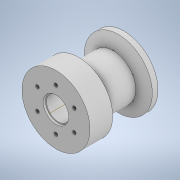
# Autodesk Inventor part: pulleyForRoundAdapter
Saved by Autodesk Inventor 2020.2 (Build 242310000, 310)
## iProperties
Created: 2020-02-15
Part Number: pulleyForRoundAdapter
Material: Generic
Document SubType Name: Modeling
Designer: robst
Density: 1 g/cm^3
Appearance: Default
Author: robst
Autodesk Inventor part; units mm, degrees
ref_plane "YZ Plane" through (0, 0, 0) normal (1, 0, 0) x (0, 1, 0)
ref_plane "XZ Plane" through (0, 0, 0) normal (0, 1, 0) x (-1, 0, 0)
ref_plane "XY Plane" through (0, 0, 0) normal (0, 0, 1) x (1, 0, 0)
sketch "Sketch1" plane through (0, 0, 0) normal (0, 0, 1) x (1, 0, 0)
  circle A0 centre (0, 0) radius 25.4
  dimension "d0" = 50.8
  constraints: 2 coincident, 1 centre point
  measures "d0" diameter of A0
extrude "Extrusion1" add sketch "Sketch1" along normal mid plane 76.2
sketch "Sketch3" plane through (0, 0, 0) normal (1, 0, 0) x (0, 1, 0)
  line L0 (25.4, 38.1) -> (-25.4, 38.1) projected
  line L1 (25.4, 38.1) -> (38.1, 38.1)
  line L2 (25.4, -38.1) -> (25.4, 38.1) projected
  line L3 (0, -53.34) -> (0, 53.34) projected
  line L4 (38.1, 38.1) -> (38.1, 12.7)
  line L5 (38.1, 12.7) -> (24.2886, 6.2597)
  line L6 (24.2886, 6.2597) -> (25.4, 6.7779)
  line L7 (25.4, -38.1) -> (25.4, 38.1) projected
  point P0 (0, 0)
  point P1 (25.4, 19.4779)
  point P2 (25.4, 6.7779)
  point P3 (25.4, 6.7779)
  dimension "d9" = 12.7
  dimension "d12" = 25.4
  dimension "d13" = 115
  constraints: 8 end point, 2 point on line, 1 collinear, 1 horizontal, 1 vertical
  measures "d9" distance of L0.start L1.end
  measures "d12" distance of L1.end L4.end
  measures "d13" angle of L4 L5
revolve "Revolution1" add sketch "Sketch3" angle 360 about axis through (0, 0, -10) along (0, 0, 1)
sketch "Sketch4" plane through (0, 0, 0) normal (1, 0, 0) x (0, 1, 0)
  line L0 (25.4, -38.1) -> (25.4, 6.7779) projected
  line L1 (-25.4, -38.1) -> (25.4, -38.1) projected
  line L2 (25.4, -38.1) -> (38.1, -38.1)
  line L3 (38.1, -38.1) -> (38.1, -31.75)
  line L4 (38.1, -31.75) -> (24.8707, -25.5811)
  line L5 (0, -46.9275) -> (0, 14.8652) projected
  line L6 (24.8707, -25.5811) -> (25.4, -25.8279)
  line L7 (25.4, -38.1) -> (25.4, 6.7779) projected
  point P0 (0, 0)
  dimension "d14" = 12.7
  dimension "d15" = 6.35
  dimension "d16" = 115
  constraints: 8 end point, 1 collinear, 1 horizontal, 1 perpendicular, 1 point on line
  measures "d14" distance of L0.start L2.end
  measures "d15" distance of L2.end L3.end
  measures "d16" angle of L4 L3
revolve "Revolution2" add sketch "Sketch4" angle 360 about axis through (0, 0, -10) along (0, 0, 1)
sketch "Sketch5" plane through (0, 0, 38.1) normal (0, 0, 1) x (1, 0, 0)
  circle A0 centre (0, 0) radius 13.0969
  dimension "d18" = 26.1938
  constraints: 1 centre point, 1 coincident
  measures "d18" diameter of A0
extrude "Extrusion4" cut sketch "Sketch5" against normal blind 25.4
sketch "Sketch6" plane through (0, 0, 38.1) normal (0, 0, 1) x (1, 0, 0)
  circle A0 centre (0, 0) radius 14.2875
  dimension "d21" = 28.575
  constraints: 1 centre point, 1 coincident
  measures "d21" diameter of A0
extrude "Extrusion5" cut sketch "Sketch6" against normal blind 2.54
mirror "Mirror2" about plane through (0, 0, 0) normal (0, 0, 1) of "Extrusion5", "Extrusion4"
sketch "Sketch8" plane through (0, 0, 38.1) normal (0, 0, 1) x (1, 0, 0)
  point P0 (0, 0)
  point P1 (0, 23.8125)
  point P2 (-20.6222, 11.9063)
  point P3 (0, 0)
  point P4 (-20.6222, -11.9062)
  point P5 (0, 0)
  point P6 (0, -23.8125)
  point P7 (0, 0)
  point P8 (20.6222, -11.9063)
  point P9 (0, 0)
  point P10 (20.6222, 11.9062)
  point P11 (0, 0)
  dimension "d32" = 23.8125
  dimension "d35" = 360
  constraints: 2 coincident, 11 other
  measures "d32" distance of point (0, 0) point (0, 23.812)
hole "Hole1" at (0, 23.8125, 38.1) at (-20.6222, 11.9063, 38.1) at (-20.6222, -11.9062, 38.1) at (0, -23.8125, 38.1) at (20.6222, -11.9063, 38.1) at (20.6222, 11.9062, 38.1) direction (0, 0, -1) diameter 3.9624 depth 13.6144 tip angle 118 thread size "10-32 UNF" class "2B" standard "ANSI Unified Screw Threads"
sketch "Sketch9" plane through (0, 0, -38.1) normal (0, 0, -1) x (-1, 0, 0)
  point P0 (0, 0)
  point P1 (0, 23.8125)
  point P2 (-20.6222, 11.9063)
  point P3 (-20.6222, -11.9062)
  point P4 (0, -23.8125)
  point P5 (20.6222, -11.9063)
  point P6 (20.6222, 11.9062)
  dimension "d44" = 23.8125
  dimension "d47" = 360
  constraints: 7 other
  measures "d44" distance of point (0, 0) point (0, 23.812)
hole "Hole2" at (0, 23.8125, -38.1) at (20.6222, 11.9063, -38.1) at (20.6222, -11.9062, -38.1) at (0, -23.8125, -38.1) at (-20.6222, -11.9063, -38.1) at (-20.6222, 11.9062, -38.1) direction (0, 0, 1) diameter 3.9624 depth 12.065 tip angle 118 thread size "10-32 UNF" class "2B" standard "ANSI Unified Screw Threads"
body "Solid1"
